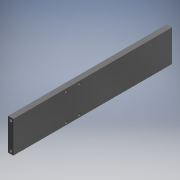
# Autodesk Inventor part: Motor mount bar
Saved by Autodesk Inventor 2019 (Build 230136000, 136)
## iProperties
Part Number: Motor mount bar
Material: Generic
Document SubType Name: Modeling
Designer: Delta
Appearance: Default
Author: Delta
Autodesk Inventor part; units mm, degrees
ref_plane "YZ Plane" through (0, 0, 0) normal (1, 0, 0) x (0, 1, 0)
ref_plane "XZ Plane" through (0, 0, 0) normal (0, 1, 0) x (-1, 0, 0)
ref_plane "XY Plane" through (0, 0, 0) normal (0, 0, 1) x (1, 0, 0)
sketch "Sketch1" plane through (0, 0, 0) normal (0, 0, 1) x (1, 0, 0)
  line L0 (0, 0) -> (6.35, 0)
  line L1 (6.35, 0) -> (6.35, 38.1)
  line L2 (6.35, 38.1) -> (0, 38.1)
  line L3 (0, 38.1) -> (0, 0)
  dimension "d0" = 6.35
  dimension "d1" = 38.1
  constraints: 8 end point, 2 parallel, 1 horizontal, 1 perpendicular
  measures "d0" distance of L2.end L1.end
  measures "d1" distance of L1.end L0.end
extrude "Extrusion1" add sketch "Sketch1" along normal blind 190.5
sketch "Sketch2" plane through (0, 0, 190.5) normal (0, 0, 1) x (1, 0, 0)
  circle A0 centre (3.175, 3.175) radius 1.651
  circle A1 centre (3.175, 34.925) radius 1.651
  line L0 (0, 38.1) -> (0, 0) projected
  line L1 (6.35, 38.1) -> (0, 38.1) projected
  line L2 (6.35, 0) -> (6.35, 38.1) projected
  line L3 (0, 0) -> (6.35, 0) projected
  dimension "d4" = 3.302
  dimension "d5" = 3.302
  dimension "d6" = 3.175
  dimension "d7" = 3.175
  dimension "d8" = 3.175
  dimension "d9" = 3.175
  constraints: 2 centre point
  measures "d4" diameter of A0
  measures "d5" diameter of A1
  measures "d6" distance from line of L0 A1.centre
  measures "d7" distance from line of L1 A1.centre
  measures "d8" distance from line of L2 A0.centre
  measures "d9" distance from line of L3 A0.centre
extrude "Extrusion2" cut sketch "Sketch2" against normal blind 6.35 contours A0 | A1
ref_plane "Work Plane1" through (0, 0, 95.25) normal (0, 0, 1) x (1, 0, 0)
mirror "Mirror1" about plane through (0, 0, 95.25) normal (0, 0, 1) of "Extrusion2"
sketch "Sketch3" plane through (0, 0, 0) normal (-1, 0, 0) x (0, 0, 1)
  line L0 (0, 0) -> (190.5, 0) projected
  line L1 (190.5, 38.1) -> (190.5, 0) projected
  line L2 (0, 38.1) -> (0, 0) projected
  circle A0 centre (110.998, 3.048) radius 1.4605
  circle A1 centre (127, 3.048) radius 1.4605
  dimension "d12" = 3.048
  dimension "d13" = 3.048
  dimension "d14" = 16.002
  dimension "d15" = 63.5
  dimension "d16" = 110.998
  dimension "d17" = 2.921
  dimension "d18" = 2.921
  constraints: 2 centre point, 2 coincident
  measures "d12" distance from line of L0 point (127, 3.048)
  measures "d13" distance from line of L0 point (110.998, 3.048)
  measures "d14" distance of point (110.998, 3.048) point (127, 3.048)
  measures "d15" distance from line of L1 point (127, 3.048)
  measures "d16" distance from line of L2 point (110.998, 3.048)
  measures "d17" diameter of A0
  measures "d18" diameter of A1
extrude "Extrusion3" cut sketch "Sketch3" against normal through all
ref_plane "Work Plane2" through (0, 19.05, 0) normal (0, 1, 0) x (1, 0, 0)
mirror "Mirror2" about plane through (0, 19.05, 0) normal (0, 1, 0) of "Extrusion3"
equation "\"d4\" = d5"
equation "\"d7\" = d6"
equation "\"d8\" = d6"
equation "\"d9\" = d6"
equation "\"d13\" = d12"
equation "\"d17\" = d18"
body "Solid1"
